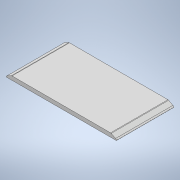
# Autodesk Inventor part: pokrywa_czołg
Saved by Autodesk Inventor 2021 (Build 250183000, 183)
## iProperties
Created: 2022-01-30
Part Number: pokrywa_czołg
Material: Generic
Document SubType Name: Modeling
Designer: Łukasz
Density: 1 g/cm^3
Appearance: Default
Author: Łukasz
Autodesk Inventor part; units mm, degrees
ref_plane "YZ Plane" through (0, 0, 0) normal (1, 0, 0) x (0, 1, 0)
ref_plane "XZ Plane" through (0, 0, 0) normal (0, 1, 0) x (-1, 0, 0)
ref_plane "XY Plane" through (0, 0, 0) normal (0, 0, 1) x (1, 0, 0)
sketch "Sketch1" plane through (0, 0, 0) normal (0, 0, 1) x (1, 0, 0)
  line L0 (328.3961, 60) -> (-3.3961, 60)
  line L1 (-3.3961, 60) -> (-22.5738, 50.2284)
  line L2 (347.5738, 50.2284) -> (328.3961, 60)
  line L3 (-22.5738, 53.5954) -> (-4.1163, 63)
  line L4 (-4.1163, 63) -> (329.1163, 63)
  line L5 (329.1163, 63) -> (347.5738, 53.5954)
  line L6 (-22.5738, 50.2284) -> (-22.5738, 53.5954)
  line L7 (347.5738, 50.2284) -> (347.5738, 53.5954)
  point P0 (0, 0)
  dimension "d0" = 3
  constraints: 16 end point, 2 vertical
  measures "d0" distance between parallel lines of L0 L4
extrude "Extrusion1" add sketch "Sketch1" along normal blind 186.8
sketch "Sketch2" plane through (0, 0, 186.8) normal (0, 0, 1) x (1, 0, 0)
  line L0 (-22.5738, 53.5954) -> (-22.5738, 50.2284) projected
  line L1 (328.3961, 60) -> (347.5738, 50.2284) projected
  line L2 (-22.5738, 50.2284) -> (347.5738, 50.2284)
  line L3 (329.1163, 63) -> (-4.1163, 63) projected
  line L4 (-4.1163, 63) -> (-22.5738, 53.5954) projected
  line L5 (347.5738, 53.5954) -> (329.1163, 63) projected
  line L6 (347.5738, 50.2284) -> (347.5738, 53.5954) projected
  point P0 (0, 0)
  constraints: 2 end point, 1 horizontal
extrude "Extrusion2" add sketch "Sketch2" along normal blind 3
sketch "Sketch3" plane through (0, 0, 0) normal (0, 0, -1) x (-1, 0, 0)
  line L0 (-328.3961, 60) -> (-347.5738, 50.2284) projected
  line L1 (22.5738, 50.2284) -> (-347.5738, 50.2284) projected
  line L2 (22.5738, 50.2284) -> (3.3961, 60) projected
  line L3 (3.3961, 60) -> (-328.3961, 60) projected
  line L4 (-347.5738, 53.5954) -> (-329.1163, 63) projected
  line L5 (-347.5738, 50.2284) -> (-347.5738, 53.5954) projected
  line L6 (-347.5738, 53.5954) -> (-329.1163, 63) projected
  line L7 (-347.5738, 50.2284) -> (-347.5738, 53.5954) projected
  line L8 (-328.3961, 60) -> (-347.5738, 50.2284) projected
  line L9 (3.3961, 60) -> (-328.3961, 60) projected
  line L10 (22.5738, 50.2284) -> (3.3961, 60) projected
  line L11 (22.5738, 53.5954) -> (22.5738, 50.2284) projected
  line L12 (4.1163, 63) -> (22.5738, 53.5954) projected
  line L13 (-329.1163, 63) -> (4.1163, 63) projected
  point P0 (0, 0)
extrude "Extrusion3" add sketch "Sketch3" along normal blind 3
fillet "Fillet1" radius 5 4 edges at (329.1163, 63, 93.4) (347.5738, 53.5954, 93.4) (-4.1163, 63, 93.4) (-22.5738, 53.5954, 93.4)
body "Solid1"
